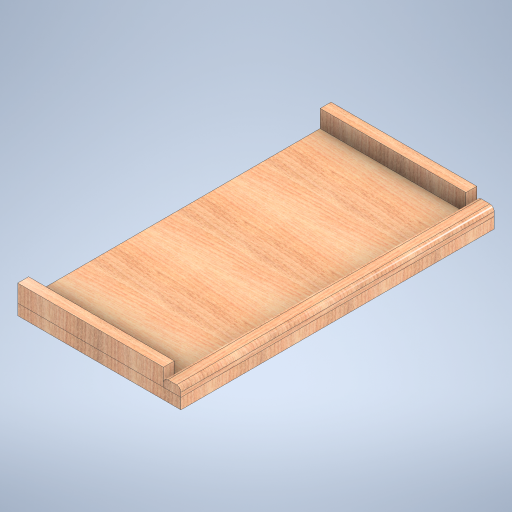
# Autodesk Inventor part: Drawer
Saved by Autodesk Inventor 2023 (Build 270158000, 158)
## iProperties
Created: 2022-09-17
Part Number: Drawer
Material: Wood (Birch)
Document SubType Name: Modeling
Designer: mliu-23
Density: 0.55 g/cm^3
Appearance: Birch - Natural Polished
Author: mliu-23
Autodesk Inventor part; units mm, degrees
ref_plane "YZ Plane" through (0, 0, 0) normal (1, 0, 0) x (0, 1, 0)
ref_plane "XZ Plane" through (0, 0, 0) normal (0, 1, 0) x (-1, 0, 0)
ref_plane "XY Plane" through (0, 0, 0) normal (0, 0, 1) x (1, 0, 0)
sketch "Sketch1" plane through (0, 0, 0) normal (0, 1, 0) x (-1, 0, 0)
  line L0 (0, 0) -> (-476.25, 0)
  line L1 (-476.25, 0) -> (-476.25, -914.4)
  line L2 (-476.25, -914.4) -> (0, -914.4)
  line L3 (0, -914.4) -> (0, 0)
  dimension "d0" = 476.25
  dimension "d1" = 914.4
  constraints: 8 end point, 2 parallel, 1 horizontal, 1 perpendicular
  measures "d0" distance of L2.end L1.end
  measures "d1" distance of L1.end L0.end
extrude "Extrusion1" add sketch "Sketch1" along normal blind 31.75
sketch "Sketch2" plane through (0, 0, 0) normal (0, 0, 1) x (1, 0, 0)
  line L0 (0, 31.75) -> (476.25, 31.75) projected
  line L1 (476.25, 0) -> (476.25, 31.75) projected
  line L2 (0, 0) -> (476.25, 0) projected
  line L3 (476.25, 0) -> (476.25, 31.75) projected
  line L4 (0, 31.75) -> (476.25, 31.75) projected
  line L5 (0, 0) -> (0, 31.75) projected
  line L6 (476.25, 31.75) -> (0, 31.75) projected
  line L7 (476.25, 31.75) -> (425.45, 31.75)
  line L8 (425.45, 31.75) -> (425.45, 57.15)
  line L9 (425.45, 57.15) -> (476.25, 57.15)
  line L10 (476.25, 57.15) -> (476.25, 31.75)
  dimension "d4" = 50.8
  dimension "d5" = 25.4
  constraints: 8 end point, 2 parallel, 1 horizontal, 1 perpendicular
  measures "d4" distance of L8.end L9.end
  measures "d5" distance of L7.end L8.end
extrude "Extrusion2" add sketch "Sketch2" against normal up to surface (914.4 mm away) separate body contours L8 L9 L10 L0
fillet "Fillet1" radius 12.7 2 edges at (476.25, 57.15, -457.2) (425.45, 57.15, -457.2)
sketch "Sketch3" plane through (0, 31.75, 0) normal (0, 1, 0) x (1, 0, 0)
  line L0 (0, 914.4) -> (0, 0) projected
  line L1 (425.45, 0) -> (425.45, 914.4) projected
  line L2 (0, 0) -> (425.45, 0)
  line L3 (425.45, 0) -> (425.45, 31.75)
  line L4 (425.45, 31.75) -> (0, 31.75)
  line L5 (0, 31.75) -> (0, 0)
  line L6 (0, 914.4) -> (425.45, 914.4)
  line L7 (425.45, 914.4) -> (425.45, 882.65)
  line L8 (425.45, 882.65) -> (0, 882.65)
  line L9 (0, 882.65) -> (0, 914.4)
  point P0 (0, 31.75)
  dimension "d9" = 31.75
  dimension "d10" = 31.75
  constraints: 16 end point, 4 parallel, 3 point on line, 2 horizontal, 2 perpendicular
  measures "d9" distance between parallel lines of L2 L4
  measures "d10" distance between parallel lines of L6 L8
extrude "Extrusion3" add sketch "Sketch3" along normal blind 50.8 separate body contours L6 L1 L8 L0 | L4 L1 L2 L0
body "Solid1"
body "Solid2"
body "Solid3"
